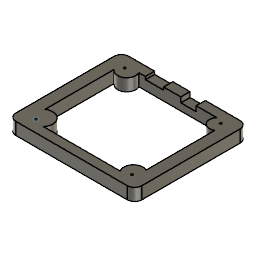
spelaro (Assembly) (Autodesk Fusion 360 design; units mm, degrees)
part number: 2026-09-10-19-06-22-338
Autodesk Fusion 360 part; units mm, degrees
sketch "Sketch2" plane through (0, 0, -0.05) normal (0, 0, -1) x (1, 0, 0)
  line L0 (260, 40) -> (153.3147, 40)
  line L1 (153.3147, 40) -> (153.3147, 134.963)
  line L2 (153.3147, 134.963) -> (260, 134.963)
  line L3 (260, 134.963) -> (260, 40)
  line L4 (254.727, 129.69) -> (254.727, 45.273)
  line L5 (254.727, 45.273) -> (158.5878, 45.273)
  line L6 (158.5878, 45.273) -> (158.5878, 129.69)
  line L7 (158.5878, 129.69) -> (254.727, 129.69)
  dimension "d1" = 5.273
  constraint horizontal L0
  constraint vertical L1
  constraint horizontal L2
  constraint vertical L3
extrude "Extrude1" add sketch "Sketch2" along normal blind 11
extrude "Extrude2" add 1 faces at (153.3147, -71.6543, -3.7167) along direction (-1, 0, 0) blind 3
extrude "Extrude3" add 1 faces at (223.4382, -40, -3.7167) along direction (0, 1, 0) blind 3
extrude "Extrude4" add 1 faces at (260, -102.3087, -3.7167) along direction (1, 0, 0) blind 3
extrude "Extrude5" add 1 faces at (225.4382, -134.963, -7.3833) along direction (0, -1, 0) blind 3
sketch "Sketch3" plane through (0, -37, 0) normal (0, 1, 0) x (-1, 0, 0)
  line L0 (-150.3147, -0.05) -> (-263, -0.05)
  line L1 (-263, -0.05) -> (-263, -11.05)
  line L2 (-263, -11.05) -> (-150.3147, -11.05)
  line L3 (-150.3147, -11.05) -> (-150.3147, -0.05)
  line L4 (-180.0368, -0.05) -> (-196.2868, -0.05)
  line L5 (-196.2868, -0.05) -> (-196.2868, -2.5147)
  line L6 (-196.2868, -2.5147) -> (-180.0368, -2.5147)
  line L7 (-180.0368, -2.5147) -> (-180.0368, -0.05)
  constraint horizontal L4
  constraint vertical L5
  constraint horizontal L6
  constraint vertical L7
  constraint coincident L0 L4.start
extrude "Extrude6" cut sketch "Sketch3" against normal blind 23 contours L0 L4 L5 L6 L7
sketch "Sketch4" plane through (0, -37, 0) normal (0, 1, 0) x (-1, 0, 0)
  line L0 (-196.2868, -2.5147) -> (-196.2868, -0.05)
  line L1 (-196.2868, -0.05) -> (-263, -0.05)
  line L2 (-263, -0.05) -> (-263, -11.05)
  line L3 (-263, -11.05) -> (-150.3147, -11.05)
  line L4 (-150.3147, -11.05) -> (-150.3147, -0.05)
  line L5 (-150.3147, -0.05) -> (-180.0368, -0.05)
  line L6 (-180.0368, -0.05) -> (-180.0368, -2.5147)
  line L7 (-180.0368, -2.5147) -> (-196.2868, -2.5147)
  line L8 (-223.6278, -0.05) -> (-213.3861, -0.05)
  line L9 (-213.3861, -0.05) -> (-213.3861, -4.6383)
  line L10 (-213.3861, -4.6383) -> (-223.6278, -4.6383)
  line L11 (-223.6278, -4.6383) -> (-223.6278, -0.05)
  constraint horizontal L8
  constraint vertical L9
  constraint horizontal L10
  constraint vertical L11
  constraint coincident L1 L8.start
extrude "Extrude7" cut sketch "Sketch4" against normal blind 15.5 contours L1 L8 L9 L10 L11
extrude "Extrude8" add 1 faces at (158.5878, -73.412, -3.7167) along direction (1, 0, 0) blind 2
extrude "Extrude9" add 1 faces at (254.727, -101.551, -3.7167) along direction (-1, 0, 0) blind 2
sketch "Sketch5" plane through (0, 0, -0.05) normal (0, 0, -1) x (1, 0, 0)
  circle A0 centre (167, 49) radius 8.0623
extrude "Extrude10" add sketch "Sketch5" along normal blind 11
sketch "Sketch6" plane through (0, 0, -0.05) normal (0, 0, -1) x (1, 0, 0)
  circle A0 centre (166, 126) radius 7.8102
  circle A1 centre (247, 125) radius 9.2195
  circle A2 centre (249, 50) radius 7.0711
extrude "Extrude11" add sketch "Sketch6" along normal blind 11 contours A2
sketch "Sketch7" plane through (0, 0, -0.05) normal (0, 0, -1) x (1, 0, 0)
  circle A0 centre (249, 125) radius 8.6023
extrude "Extrude12" add sketch "Sketch7" along normal blind 11
sketch "Sketch8" plane through (0, 0, -0.05) normal (0, 0, -1) x (1, 0, 0)
  circle A0 centre (165.8963, 123.5709) radius 9.6029
extrude "Extrude13" add sketch "Sketch8" along normal blind 11
fillet "Fillet1" radius 6.5 1 edges at (263, -137.963, -5.55)
fillet "Fillet2" radius 6.5 1 edges at (263, -37, -5.55)
fillet "Fillet3" radius 6.5 1 edges at (150.3147, -37, -5.55)
fillet "Fillet4" radius 6.5 1 edges at (150.3147, -137.963, -5.55)
sketch "Sketch9" plane through (0, 0, 0) normal (0, 0, 1) x (-1, 0, 0)
  circle A0 centre (-164.22, 127.34) radius 2.2
  circle A1 centre (-165.3867, 128.5067) radius 0.175
  circle A2 centre (-164.22, 128.99) radius 0.175
  circle A3 centre (-165.87, 127.34) radius 0.175
  circle A4 centre (-164.22, 127.34) radius 1.075
  circle A5 centre (-163.0533, 128.5067) radius 0.175
  circle A6 centre (-162.57, 127.34) radius 0.175
  circle A7 centre (-165.3867, 126.1733) radius 0.175
  circle A8 centre (-164.22, 125.69) radius 0.175
  circle A9 centre (-163.0533, 126.1733) radius 0.175
sketch "Sketch10" plane through (0, 0, 1.56) normal (0, 0, 1) x (-1, 0, 0)
  arc A0 (-164.0236, 44.0124) -> (-160.2224, 47.8136) centre (-164.22, 48.01) ccw
  line L0 (-160.2224, 47.8136) -> (-160.22, 48.01)
  line L1 (-160.22, 48.01) -> (-160.22, 127.34)
  line L2 (-160.22, 127.34) -> (-160.2224, 127.5364)
  arc A1 (-160.2224, 127.5364) -> (-164.0236, 131.3376) centre (-164.22, 127.34) ccw
  line L3 (-164.0236, 131.3376) -> (-164.22, 131.34)
  line L4 (-164.22, 131.34) -> (-250.06, 131.34)
  line L5 (-250.06, 131.34) -> (-250.2564, 131.3376)
  arc A2 (-250.2564, 131.3376) -> (-254.0576, 127.5364) centre (-250.06, 127.34) ccw
  line L6 (-254.0576, 127.5364) -> (-254.06, 127.34)
  line L7 (-254.06, 127.34) -> (-254.06, 48.01)
  line L8 (-254.06, 48.01) -> (-254.0576, 47.8136)
  arc A3 (-254.0576, 47.8136) -> (-250.2564, 44.0124) centre (-250.06, 48.01) ccw
  line L9 (-250.2564, 44.0124) -> (-250.06, 44.01)
  line L10 (-250.06, 44.01) -> (-164.22, 44.01)
  line L11 (-164.22, 44.01) -> (-164.0236, 44.0124)
  circle A4 centre (-164.22, 127.34) radius 2.2
  circle A5 centre (-250.06, 127.34) radius 2.2
  circle A6 centre (-188.38, 126.32) radius 1.1
  circle A7 centre (-198.58, 126.32) radius 1.1
  arc A8 (-214.77, 126.55) -> (-214.77, 124.65) centre (-214.77, 125.6) ccw
  line L12 (-214.77, 126.55) -> (-213.47, 126.55)
  arc A9 (-213.47, 124.65) -> (-213.47, 126.55) centre (-213.47, 125.6) ccw
  line L13 (-213.47, 124.65) -> (-214.77, 124.65)
  arc A10 (-227.27, 126.55) -> (-227.27, 124.65) centre (-227.27, 125.6) ccw
  line L14 (-227.27, 126.55) -> (-225.97, 126.55)
  arc A11 (-225.97, 124.65) -> (-225.97, 126.55) centre (-225.97, 125.6) ccw
  line L15 (-225.97, 124.65) -> (-227.27, 124.65)
  circle A12 centre (-188.38, 123.57) radius 0.9
  circle A13 centre (-198.58, 123.57) radius 0.9
  arc A14 (-214.77, 121.55) -> (-214.77, 119.65) centre (-214.77, 120.6) ccw
  line L16 (-214.77, 121.55) -> (-213.47, 121.55)
  arc A15 (-213.47, 119.65) -> (-213.47, 121.55) centre (-213.47, 120.6) ccw
  line L17 (-213.47, 119.65) -> (-214.77, 119.65)
  arc A16 (-227.27, 121.55) -> (-227.27, 119.65) centre (-227.27, 120.6) ccw
  line L18 (-227.27, 121.55) -> (-225.97, 121.55)
  arc A17 (-225.97, 119.65) -> (-225.97, 121.55) centre (-225.97, 120.6) ccw
  line L19 (-225.97, 119.65) -> (-227.27, 119.65)
  circle A18 centre (-188.38, 119.92) radius 1.1
  circle A19 centre (-198.58, 119.92) radius 1.1
  circle A20 centre (-248.26, 102) radius 0.85
  circle A21 centre (-248.26, 99.46) radius 0.85
  circle A22 centre (-248.26, 96.92) radius 0.85
  circle A23 centre (-248.26, 94.38) radius 0.85
  circle A24 centre (-248.26, 91.84) radius 0.85
  circle A25 centre (-248.26, 89.3) radius 0.85
  circle A26 centre (-248.26, 86.76) radius 0.85
  circle A27 centre (-248.26, 84.22) radius 0.85
  circle A28 centre (-248.26, 81.68) radius 0.85
  circle A29 centre (-248.26, 79.14) radius 0.85
  circle A30 centre (-248.26, 76.6) radius 0.85
  circle A31 centre (-248.26, 74.06) radius 0.85
  circle A32 centre (-248.26, 71.52) radius 0.85
  line L20 (-249.11, 68.13) -> (-249.11, 69.83)
  line L21 (-249.11, 69.83) -> (-247.41, 69.83)
  line L22 (-247.41, 69.83) -> (-247.41, 68.13)
  line L23 (-247.41, 68.13) -> (-249.11, 68.13)
  circle A33 centre (-202.95, 54.5201) radius 0.6604
  circle A34 centre (-205.49, 54.5201) radius 0.6604
  circle A35 centre (-208.03, 54.5201) radius 0.6604
  arc A36 (-215.57, 49.8) -> (-216.67, 49.8) centre (-216.12, 49.8) ccw
  line L24 (-215.57, 49.8) -> (-215.57, 49.4)
  arc A37 (-216.67, 49.4) -> (-215.57, 49.4) centre (-216.12, 49.4) ccw
  line L25 (-216.67, 49.4) -> (-216.67, 49.8)
  arc A38 (-220.41, 49.8) -> (-221.51, 49.8) centre (-220.96, 49.8) ccw
  line L26 (-220.41, 49.8) -> (-220.41, 49.4)
  arc A39 (-221.51, 49.4) -> (-220.41, 49.4) centre (-220.96, 49.4) ccw
  line L27 (-221.51, 49.4) -> (-221.51, 49.8)
  circle A40 centre (-164.22, 48.01) radius 2.2
  circle A41 centre (-250.06, 48.01) radius 2.2
  arc A42 (-215.1383, 46.8412) -> (-216.485, 46.775) centre (-215.81, 46.775) ccw
  line L28 (-215.1383, 46.8412) -> (-215.135, 46.425)
  arc A43 (-216.4817, 46.3588) -> (-215.135, 46.425) centre (-215.81, 46.425) ccw
  line L29 (-216.4817, 46.3588) -> (-216.485, 46.775)
  arc A44 (-220.5983, 46.8412) -> (-221.945, 46.775) centre (-221.27, 46.775) ccw
  line L30 (-220.5983, 46.8412) -> (-220.595, 46.425)
  arc A45 (-221.9417, 46.3588) -> (-220.595, 46.425) centre (-221.27, 46.425) ccw
  line L31 (-221.9417, 46.3588) -> (-221.945, 46.775)
  circle A46 centre (-164.22, 48.01) radius 0.9003
  constraint concentric A0 A46
extrude "Extrude14" cut sketch "Sketch10" against normal blind 13 contours A46
sketch "Sketch11" plane through (0, 0, 1.56) normal (0, 0, 1) x (-1, 0, 0)
  arc A0 (-164.0236, 44.0124) -> (-160.2224, 47.8136) centre (-164.22, 48.01) ccw
  line L0 (-160.2224, 47.8136) -> (-160.22, 48.01)
  line L1 (-160.22, 48.01) -> (-160.22, 127.34)
  line L2 (-160.22, 127.34) -> (-160.2224, 127.5364)
  arc A1 (-160.2224, 127.5364) -> (-164.0236, 131.3376) centre (-164.22, 127.34) ccw
  line L3 (-164.0236, 131.3376) -> (-164.22, 131.34)
  line L4 (-164.22, 131.34) -> (-250.06, 131.34)
  line L5 (-250.06, 131.34) -> (-250.2564, 131.3376)
  arc A2 (-250.2564, 131.3376) -> (-254.0576, 127.5364) centre (-250.06, 127.34) ccw
  line L6 (-254.0576, 127.5364) -> (-254.06, 127.34)
  line L7 (-254.06, 127.34) -> (-254.06, 48.01)
  line L8 (-254.06, 48.01) -> (-254.0576, 47.8136)
  arc A3 (-254.0576, 47.8136) -> (-250.2564, 44.0124) centre (-250.06, 48.01) ccw
  line L9 (-250.2564, 44.0124) -> (-250.06, 44.01)
  line L10 (-250.06, 44.01) -> (-164.22, 44.01)
  line L11 (-164.22, 44.01) -> (-164.0236, 44.0124)
  circle A4 centre (-164.22, 127.34) radius 2.2
  circle A5 centre (-250.06, 127.34) radius 2.2
  circle A6 centre (-188.38, 126.32) radius 1.1
  circle A7 centre (-198.58, 126.32) radius 1.1
  arc A8 (-214.77, 126.55) -> (-214.77, 124.65) centre (-214.77, 125.6) ccw
  line L12 (-214.77, 126.55) -> (-213.47, 126.55)
  arc A9 (-213.47, 124.65) -> (-213.47, 126.55) centre (-213.47, 125.6) ccw
  line L13 (-213.47, 124.65) -> (-214.77, 124.65)
  arc A10 (-227.27, 126.55) -> (-227.27, 124.65) centre (-227.27, 125.6) ccw
  line L14 (-227.27, 126.55) -> (-225.97, 126.55)
  arc A11 (-225.97, 124.65) -> (-225.97, 126.55) centre (-225.97, 125.6) ccw
  line L15 (-225.97, 124.65) -> (-227.27, 124.65)
  circle A12 centre (-188.38, 123.57) radius 0.9
  circle A13 centre (-198.58, 123.57) radius 0.9
  arc A14 (-214.77, 121.55) -> (-214.77, 119.65) centre (-214.77, 120.6) ccw
  line L16 (-214.77, 121.55) -> (-213.47, 121.55)
  arc A15 (-213.47, 119.65) -> (-213.47, 121.55) centre (-213.47, 120.6) ccw
  line L17 (-213.47, 119.65) -> (-214.77, 119.65)
  arc A16 (-227.27, 121.55) -> (-227.27, 119.65) centre (-227.27, 120.6) ccw
  line L18 (-227.27, 121.55) -> (-225.97, 121.55)
  arc A17 (-225.97, 119.65) -> (-225.97, 121.55) centre (-225.97, 120.6) ccw
  line L19 (-225.97, 119.65) -> (-227.27, 119.65)
  circle A18 centre (-188.38, 119.92) radius 1.1
  circle A19 centre (-198.58, 119.92) radius 1.1
  circle A20 centre (-248.26, 102) radius 0.85
  circle A21 centre (-248.26, 99.46) radius 0.85
  circle A22 centre (-248.26, 96.92) radius 0.85
  circle A23 centre (-248.26, 94.38) radius 0.85
  circle A24 centre (-248.26, 91.84) radius 0.85
  circle A25 centre (-248.26, 89.3) radius 0.85
  circle A26 centre (-248.26, 86.76) radius 0.85
  circle A27 centre (-248.26, 84.22) radius 0.85
  circle A28 centre (-248.26, 81.68) radius 0.85
  circle A29 centre (-248.26, 79.14) radius 0.85
  circle A30 centre (-248.26, 76.6) radius 0.85
  circle A31 centre (-248.26, 74.06) radius 0.85
  circle A32 centre (-248.26, 71.52) radius 0.85
  line L20 (-249.11, 68.13) -> (-249.11, 69.83)
  line L21 (-249.11, 69.83) -> (-247.41, 69.83)
  line L22 (-247.41, 69.83) -> (-247.41, 68.13)
  line L23 (-247.41, 68.13) -> (-249.11, 68.13)
  circle A33 centre (-202.95, 54.5201) radius 0.6604
  circle A34 centre (-205.49, 54.5201) radius 0.6604
  circle A35 centre (-208.03, 54.5201) radius 0.6604
  arc A36 (-215.57, 49.8) -> (-216.67, 49.8) centre (-216.12, 49.8) ccw
  line L24 (-215.57, 49.8) -> (-215.57, 49.4)
  arc A37 (-216.67, 49.4) -> (-215.57, 49.4) centre (-216.12, 49.4) ccw
  line L25 (-216.67, 49.4) -> (-216.67, 49.8)
  arc A38 (-220.41, 49.8) -> (-221.51, 49.8) centre (-220.96, 49.8) ccw
  line L26 (-220.41, 49.8) -> (-220.41, 49.4)
  arc A39 (-221.51, 49.4) -> (-220.41, 49.4) centre (-220.96, 49.4) ccw
  line L27 (-221.51, 49.4) -> (-221.51, 49.8)
  circle A40 centre (-164.22, 48.01) radius 2.2
  circle A41 centre (-250.06, 48.01) radius 2.2
  arc A42 (-215.1383, 46.8412) -> (-216.485, 46.775) centre (-215.81, 46.775) ccw
  line L28 (-215.1383, 46.8412) -> (-215.135, 46.425)
  arc A43 (-216.4817, 46.3588) -> (-215.135, 46.425) centre (-215.81, 46.425) ccw
  line L29 (-216.4817, 46.3588) -> (-216.485, 46.775)
  arc A44 (-220.5983, 46.8412) -> (-221.945, 46.775) centre (-221.27, 46.775) ccw
  line L30 (-220.5983, 46.8412) -> (-220.595, 46.425)
  arc A45 (-221.9417, 46.3588) -> (-220.595, 46.425) centre (-221.27, 46.425) ccw
  line L31 (-221.9417, 46.3588) -> (-221.945, 46.775)
  circle A46 centre (-250.06, 48.01) radius 0.9005
  dimension "d38" = 1.801
  constraint concentric A3 A46
  measures "d38" diameter of A46
extrude "Extrude15" cut sketch "Sketch11" against normal blind 14 contours A46
sketch "Sketch12" plane through (0, 0, 1.56) normal (0, 0, 1) x (-1, 0, 0)
  arc A0 (-164.0236, 44.0124) -> (-160.2224, 47.8136) centre (-164.22, 48.01) ccw
  line L0 (-160.2224, 47.8136) -> (-160.22, 48.01)
  line L1 (-160.22, 48.01) -> (-160.22, 127.34)
  line L2 (-160.22, 127.34) -> (-160.2224, 127.5364)
  arc A1 (-160.2224, 127.5364) -> (-164.0236, 131.3376) centre (-164.22, 127.34) ccw
  line L3 (-164.0236, 131.3376) -> (-164.22, 131.34)
  line L4 (-164.22, 131.34) -> (-250.06, 131.34)
  line L5 (-250.06, 131.34) -> (-250.2564, 131.3376)
  arc A2 (-250.2564, 131.3376) -> (-254.0576, 127.5364) centre (-250.06, 127.34) ccw
  line L6 (-254.0576, 127.5364) -> (-254.06, 127.34)
  line L7 (-254.06, 127.34) -> (-254.06, 48.01)
  line L8 (-254.06, 48.01) -> (-254.0576, 47.8136)
  arc A3 (-254.0576, 47.8136) -> (-250.2564, 44.0124) centre (-250.06, 48.01) ccw
  line L9 (-250.2564, 44.0124) -> (-250.06, 44.01)
  line L10 (-250.06, 44.01) -> (-164.22, 44.01)
  line L11 (-164.22, 44.01) -> (-164.0236, 44.0124)
  circle A4 centre (-164.22, 127.34) radius 2.2
  circle A5 centre (-250.06, 127.34) radius 2.2
  circle A6 centre (-188.38, 126.32) radius 1.1
  circle A7 centre (-198.58, 126.32) radius 1.1
  arc A8 (-214.77, 126.55) -> (-214.77, 124.65) centre (-214.77, 125.6) ccw
  line L12 (-214.77, 126.55) -> (-213.47, 126.55)
  arc A9 (-213.47, 124.65) -> (-213.47, 126.55) centre (-213.47, 125.6) ccw
  line L13 (-213.47, 124.65) -> (-214.77, 124.65)
  arc A10 (-227.27, 126.55) -> (-227.27, 124.65) centre (-227.27, 125.6) ccw
  line L14 (-227.27, 126.55) -> (-225.97, 126.55)
  arc A11 (-225.97, 124.65) -> (-225.97, 126.55) centre (-225.97, 125.6) ccw
  line L15 (-225.97, 124.65) -> (-227.27, 124.65)
  circle A12 centre (-188.38, 123.57) radius 0.9
  circle A13 centre (-198.58, 123.57) radius 0.9
  arc A14 (-214.77, 121.55) -> (-214.77, 119.65) centre (-214.77, 120.6) ccw
  line L16 (-214.77, 121.55) -> (-213.47, 121.55)
  arc A15 (-213.47, 119.65) -> (-213.47, 121.55) centre (-213.47, 120.6) ccw
  line L17 (-213.47, 119.65) -> (-214.77, 119.65)
  arc A16 (-227.27, 121.55) -> (-227.27, 119.65) centre (-227.27, 120.6) ccw
  line L18 (-227.27, 121.55) -> (-225.97, 121.55)
  arc A17 (-225.97, 119.65) -> (-225.97, 121.55) centre (-225.97, 120.6) ccw
  line L19 (-225.97, 119.65) -> (-227.27, 119.65)
  circle A18 centre (-188.38, 119.92) radius 1.1
  circle A19 centre (-198.58, 119.92) radius 1.1
  circle A20 centre (-248.26, 102) radius 0.85
  circle A21 centre (-248.26, 99.46) radius 0.85
  circle A22 centre (-248.26, 96.92) radius 0.85
  circle A23 centre (-248.26, 94.38) radius 0.85
  circle A24 centre (-248.26, 91.84) radius 0.85
  circle A25 centre (-248.26, 89.3) radius 0.85
  circle A26 centre (-248.26, 86.76) radius 0.85
  circle A27 centre (-248.26, 84.22) radius 0.85
  circle A28 centre (-248.26, 81.68) radius 0.85
  circle A29 centre (-248.26, 79.14) radius 0.85
  circle A30 centre (-248.26, 76.6) radius 0.85
  circle A31 centre (-248.26, 74.06) radius 0.85
  circle A32 centre (-248.26, 71.52) radius 0.85
  line L20 (-249.11, 68.13) -> (-249.11, 69.83)
  line L21 (-249.11, 69.83) -> (-247.41, 69.83)
  line L22 (-247.41, 69.83) -> (-247.41, 68.13)
  line L23 (-247.41, 68.13) -> (-249.11, 68.13)
  circle A33 centre (-202.95, 54.5201) radius 0.6604
  circle A34 centre (-205.49, 54.5201) radius 0.6604
  circle A35 centre (-208.03, 54.5201) radius 0.6604
  arc A36 (-215.57, 49.8) -> (-216.67, 49.8) centre (-216.12, 49.8) ccw
  line L24 (-215.57, 49.8) -> (-215.57, 49.4)
  arc A37 (-216.67, 49.4) -> (-215.57, 49.4) centre (-216.12, 49.4) ccw
  line L25 (-216.67, 49.4) -> (-216.67, 49.8)
  arc A38 (-220.41, 49.8) -> (-221.51, 49.8) centre (-220.96, 49.8) ccw
  line L26 (-220.41, 49.8) -> (-220.41, 49.4)
  arc A39 (-221.51, 49.4) -> (-220.41, 49.4) centre (-220.96, 49.4) ccw
  line L27 (-221.51, 49.4) -> (-221.51, 49.8)
  circle A40 centre (-164.22, 48.01) radius 2.2
  circle A41 centre (-250.06, 48.01) radius 2.2
  arc A42 (-215.1383, 46.8412) -> (-216.485, 46.775) centre (-215.81, 46.775) ccw
  line L28 (-215.1383, 46.8412) -> (-215.135, 46.425)
  arc A43 (-216.4817, 46.3588) -> (-215.135, 46.425) centre (-215.81, 46.425) ccw
  line L29 (-216.4817, 46.3588) -> (-216.485, 46.775)
  arc A44 (-220.5983, 46.8412) -> (-221.945, 46.775) centre (-221.27, 46.775) ccw
  line L30 (-220.5983, 46.8412) -> (-220.595, 46.425)
  arc A45 (-221.9417, 46.3588) -> (-220.595, 46.425) centre (-221.27, 46.425) ccw
  line L31 (-221.9417, 46.3588) -> (-221.945, 46.775)
  circle A46 centre (-250.06, 127.34) radius 0.9005
  dimension "d41" = 1.801
  constraint concentric A2 A46
  measures "d41" diameter of A46
extrude "Extrude16" cut sketch "Sketch12" against normal blind 13 contours A46
sketch "Sketch13" plane through (0, 0, 1.56) normal (0, 0, 1) x (-1, 0, 0)
  arc A0 (-164.0236, 44.0124) -> (-160.2224, 47.8136) centre (-164.22, 48.01) ccw
  line L0 (-160.2224, 47.8136) -> (-160.22, 48.01)
  line L1 (-160.22, 48.01) -> (-160.22, 127.34)
  line L2 (-160.22, 127.34) -> (-160.2224, 127.5364)
  arc A1 (-160.2224, 127.5364) -> (-164.0236, 131.3376) centre (-164.22, 127.34) ccw
  line L3 (-164.0236, 131.3376) -> (-164.22, 131.34)
  line L4 (-164.22, 131.34) -> (-250.06, 131.34)
  line L5 (-250.06, 131.34) -> (-250.2564, 131.3376)
  arc A2 (-250.2564, 131.3376) -> (-254.0576, 127.5364) centre (-250.06, 127.34) ccw
  line L6 (-254.0576, 127.5364) -> (-254.06, 127.34)
  line L7 (-254.06, 127.34) -> (-254.06, 48.01)
  line L8 (-254.06, 48.01) -> (-254.0576, 47.8136)
  arc A3 (-254.0576, 47.8136) -> (-250.2564, 44.0124) centre (-250.06, 48.01) ccw
  line L9 (-250.2564, 44.0124) -> (-250.06, 44.01)
  line L10 (-250.06, 44.01) -> (-164.22, 44.01)
  line L11 (-164.22, 44.01) -> (-164.0236, 44.0124)
  circle A4 centre (-164.22, 127.34) radius 2.2
  circle A5 centre (-250.06, 127.34) radius 2.2
  circle A6 centre (-188.38, 126.32) radius 1.1
  circle A7 centre (-198.58, 126.32) radius 1.1
  arc A8 (-214.77, 126.55) -> (-214.77, 124.65) centre (-214.77, 125.6) ccw
  line L12 (-214.77, 126.55) -> (-213.47, 126.55)
  arc A9 (-213.47, 124.65) -> (-213.47, 126.55) centre (-213.47, 125.6) ccw
  line L13 (-213.47, 124.65) -> (-214.77, 124.65)
  arc A10 (-227.27, 126.55) -> (-227.27, 124.65) centre (-227.27, 125.6) ccw
  line L14 (-227.27, 126.55) -> (-225.97, 126.55)
  arc A11 (-225.97, 124.65) -> (-225.97, 126.55) centre (-225.97, 125.6) ccw
  line L15 (-225.97, 124.65) -> (-227.27, 124.65)
  circle A12 centre (-188.38, 123.57) radius 0.9
  circle A13 centre (-198.58, 123.57) radius 0.9
  arc A14 (-214.77, 121.55) -> (-214.77, 119.65) centre (-214.77, 120.6) ccw
  line L16 (-214.77, 121.55) -> (-213.47, 121.55)
  arc A15 (-213.47, 119.65) -> (-213.47, 121.55) centre (-213.47, 120.6) ccw
  line L17 (-213.47, 119.65) -> (-214.77, 119.65)
  arc A16 (-227.27, 121.55) -> (-227.27, 119.65) centre (-227.27, 120.6) ccw
  line L18 (-227.27, 121.55) -> (-225.97, 121.55)
  arc A17 (-225.97, 119.65) -> (-225.97, 121.55) centre (-225.97, 120.6) ccw
  line L19 (-225.97, 119.65) -> (-227.27, 119.65)
  circle A18 centre (-188.38, 119.92) radius 1.1
  circle A19 centre (-198.58, 119.92) radius 1.1
  circle A20 centre (-248.26, 102) radius 0.85
  circle A21 centre (-248.26, 99.46) radius 0.85
  circle A22 centre (-248.26, 96.92) radius 0.85
  circle A23 centre (-248.26, 94.38) radius 0.85
  circle A24 centre (-248.26, 91.84) radius 0.85
  circle A25 centre (-248.26, 89.3) radius 0.85
  circle A26 centre (-248.26, 86.76) radius 0.85
  circle A27 centre (-248.26, 84.22) radius 0.85
  circle A28 centre (-248.26, 81.68) radius 0.85
  circle A29 centre (-248.26, 79.14) radius 0.85
  circle A30 centre (-248.26, 76.6) radius 0.85
  circle A31 centre (-248.26, 74.06) radius 0.85
  circle A32 centre (-248.26, 71.52) radius 0.85
  line L20 (-249.11, 68.13) -> (-249.11, 69.83)
  line L21 (-249.11, 69.83) -> (-247.41, 69.83)
  line L22 (-247.41, 69.83) -> (-247.41, 68.13)
  line L23 (-247.41, 68.13) -> (-249.11, 68.13)
  circle A33 centre (-202.95, 54.5201) radius 0.6604
  circle A34 centre (-205.49, 54.5201) radius 0.6604
  circle A35 centre (-208.03, 54.5201) radius 0.6604
  arc A36 (-215.57, 49.8) -> (-216.67, 49.8) centre (-216.12, 49.8) ccw
  line L24 (-215.57, 49.8) -> (-215.57, 49.4)
  arc A37 (-216.67, 49.4) -> (-215.57, 49.4) centre (-216.12, 49.4) ccw
  line L25 (-216.67, 49.4) -> (-216.67, 49.8)
  arc A38 (-220.41, 49.8) -> (-221.51, 49.8) centre (-220.96, 49.8) ccw
  line L26 (-220.41, 49.8) -> (-220.41, 49.4)
  arc A39 (-221.51, 49.4) -> (-220.41, 49.4) centre (-220.96, 49.4) ccw
  line L27 (-221.51, 49.4) -> (-221.51, 49.8)
  circle A40 centre (-164.22, 48.01) radius 2.2
  circle A41 centre (-250.06, 48.01) radius 2.2
  arc A42 (-215.1383, 46.8412) -> (-216.485, 46.775) centre (-215.81, 46.775) ccw
  line L28 (-215.1383, 46.8412) -> (-215.135, 46.425)
  arc A43 (-216.4817, 46.3588) -> (-215.135, 46.425) centre (-215.81, 46.425) ccw
  line L29 (-216.4817, 46.3588) -> (-216.485, 46.775)
  arc A44 (-220.5983, 46.8412) -> (-221.945, 46.775) centre (-221.27, 46.775) ccw
  line L30 (-220.5983, 46.8412) -> (-220.595, 46.425)
  arc A45 (-221.9417, 46.3588) -> (-220.595, 46.425) centre (-221.27, 46.425) ccw
  line L31 (-221.9417, 46.3588) -> (-221.945, 46.775)
  circle A46 centre (-164.22, 127.34) radius 0.9005
  dimension "d44" = 1.801
  constraint concentric A1 A46
  measures "d44" diameter of A46
extrude "Extrude17" cut sketch "Sketch13" against normal blind 15 contours A46
sketch "Sketch14" plane through (0, -37, 0) normal (0, 1, 0) x (-1, 0, 0)
  line L0 (-156.8147, -11.05) -> (-156.8147, -0.05)
  line L1 (-156.8147, -0.05) -> (-180.0368, -0.05)
  line L2 (-180.0368, -0.05) -> (-180.0368, -2.5147)
  line L3 (-180.0368, -2.5147) -> (-196.2868, -2.5147)
  line L4 (-196.2868, -2.5147) -> (-196.2868, -0.05)
  line L5 (-196.2868, -0.05) -> (-213.3861, -0.05)
  line L6 (-213.3861, -0.05) -> (-213.3861, -4.6383)
  line L7 (-213.3861, -4.6383) -> (-223.6278, -4.6383)
  line L8 (-223.6278, -4.6383) -> (-223.6278, -0.05)
  line L9 (-223.6278, -0.05) -> (-256.5, -0.05)
  line L10 (-256.5, -0.05) -> (-256.5, -11.05)
  line L11 (-256.5, -11.05) -> (-156.8147, -11.05)
  line L12 (-223.6278, -4.6383) -> (-225.3189, -4.6383)
  line L13 (-225.3189, -4.6383) -> (-225.3189, -0.05)
  line L14 (-225.3189, -0.05) -> (-223.6278, -0.05)
  line L15 (-223.6278, -0.05) -> (-223.6278, -4.6383)
  constraint horizontal L12
  constraint vertical L13
  constraint horizontal L14
  constraint vertical L15
  constraint coincident L9 L13.end
  constraint coincident L7.end L8.start
extrude "Extrude18" cut sketch "Sketch14" against normal blind 9.5 contours L8 L9 L12 L13 L14 L15
sketch "Sketch15" plane through (0, -37, 0) normal (0, 1, 0) x (-1, 0, 0)
  line L0 (-213.3861, -4.6383) -> (-225.3189, -4.6383)
  line L1 (-225.3189, -4.6383) -> (-225.3189, -0.05)
  line L2 (-225.3189, -0.05) -> (-256.5, -0.05)
  line L3 (-256.5, -0.05) -> (-256.5, -11.05)
  line L4 (-256.5, -11.05) -> (-156.8147, -11.05)
  line L5 (-156.8147, -11.05) -> (-156.8147, -0.05)
  line L6 (-156.8147, -0.05) -> (-180.0368, -0.05)
  line L7 (-180.0368, -0.05) -> (-180.0368, -2.5147)
  line L8 (-180.0368, -2.5147) -> (-196.2868, -2.5147)
  line L9 (-196.2868, -2.5147) -> (-196.2868, -0.05)
  line L10 (-196.2868, -0.05) -> (-213.3861, -0.05)
  line L11 (-213.3861, -0.05) -> (-213.3861, -4.6383)
  line L12 (-213.3861, -4.6383) -> (-211.6951, -4.6383)
  line L13 (-211.6951, -4.6383) -> (-211.6951, -0.05)
  line L14 (-211.6951, -0.05) -> (-213.3861, -0.05)
  line L15 (-213.3861, -0.05) -> (-213.3861, -4.6383)
  constraint horizontal L12
  constraint vertical L13
  constraint horizontal L14
  constraint vertical L15
  constraint coincident L10 L13.end
  constraint coincident L0.start L11.end
extrude "Extrude19" cut sketch "Sketch15" against normal blind 9 contours L10 L11 L12 L13 L14 L15
